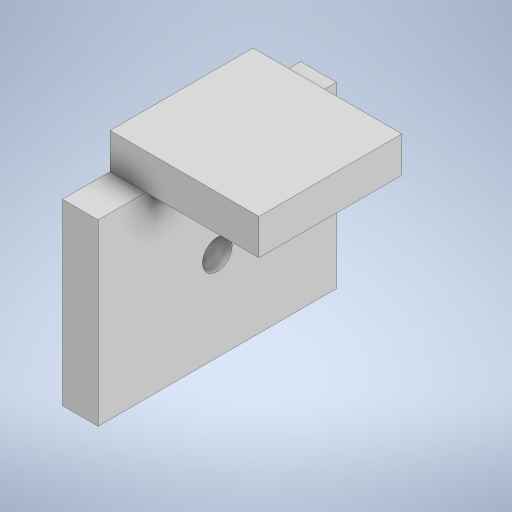
# Autodesk Inventor part: latch
Saved by Autodesk Inventor 2024 (Build 280153000, 153)
## iProperties
Created: 2024-07-03
Part Number: latch
Material: 일반
Document SubType Name: Modeling
Designer: Gihyeok Na
Density: 1 g/cm^3
Appearance: 기본값
Author: Gihyeok Na
Autodesk Inventor part; units mm, degrees
ref_plane "YZ Plane" through (0, 0, 0) normal (1, 0, 0) x (0, 1, 0)
ref_plane "XZ Plane" through (0, 0, 0) normal (0, 1, 0) x (-1, 0, 0)
ref_plane "XY Plane" through (0, 0, 0) normal (0, 0, 1) x (1, 0, 0)
sketch "스케치1" plane through (0, 0, 0) normal (1, 0, 0) x (0, 1, 0)
  line L0 (-7.5, 10) -> (7.5, 10)
  line L1 (7.5, 10) -> (7.5, -10)
  line L2 (7.5, -10) -> (-7.5, -10)
  line L3 (-7.5, -10) -> (-7.5, 10)
  line L4 (-7.5, 10) -> (7.5, -10) construction
  line L5 (7.5, 10) -> (-7.5, -10) construction
  circle A0 centre (0, 0) radius 1.25
  line L6 (7.5, 10) -> (7.5, -10)
  line L7 (7.5, -10) -> (10.5, -10)
  line L8 (10.5, -10) -> (10.5, 10)
  line L9 (10.5, 10) -> (7.5, 10)
  line L10 (10.5, -6) -> (7.5, -6)
  line L11 (10.5, 6) -> (7.5, 6)
  dimension "d0" = 15
  dimension "d1" = 20
  dimension "d2" = 2.5
  dimension "d5" = 3
  dimension "d6" = 6
  dimension "d7" = 6
  constraints: 24 end point, 4 midpoint, 4 parallel, 4 perpendicular, 4 point on line, 1 centre point, 1 coincident, 1 horizontal
  measures "d0" distance of L0.start L0.end
  measures "d1" distance of L0.end L1.end
  measures "d2" diameter of A0
  measures "d5" distance of L7.end L1.end
  measures "d6" distance from line of point (0, 0) L10
  measures "d7" distance from line of point (0, 0) L11
extrude "돌출1" add sketch "스케치1" along normal blind 3 contours L0 L1 L2 L3
extrude "돌출2" add sketch "스케치1" along normal blind 12.5 contours L11 L8 L10 L1
